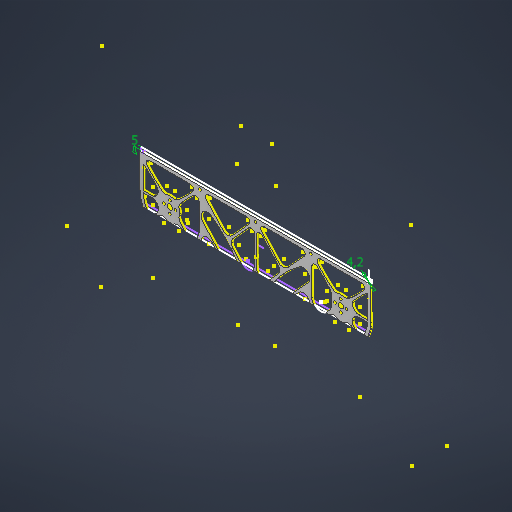
# Autodesk Inventor part: кб 2025-2026
Saved by Autodesk Inventor 2025 (Build 290162000, 162)
## iProperties
Created: 2025-09-02
Part Number: кб 2025-2026
Material: Типовые
Document SubType Name: Modeling
Designer: Phantom
Density: 1 g/cm^3
Appearance: По умолчанию
Author: Phantom
Autodesk Inventor part; units mm, degrees
(part 1 of 3)
ref_plane "YZ Plane" through (0, 0, 0) normal (1, 0, 0) x (0, 1, 0)
ref_plane "XZ Plane" through (0, 0, 0) normal (0, 1, 0) x (-1, 0, 0)
ref_plane "XY Plane" through (0, 0, 0) normal (0, 0, 1) x (1, 0, 0)
sketch "Эскиз1" plane through (0, 0, 0) normal (0, 0, 1) x (1, 0, 0)
  arc A0 (132.2862, -52.3121) -> (184.2862, -0.3121) centre (132.2862, -0.3121) ccw
  line L0 (-134.5611, -52.3121) -> (132.2862, -52.3121)
  line L1 (-186.5611, -0.3121) -> (-186.5611, 46.6879)
  line L2 (184.2862, -0.3121) -> (184.2862, 46.6879)
  line L3 (-134.5611, 51.6879) -> (-181.5611, 51.6879)
  line L4 (-181.5611, 51.6879) -> (179.2862, 51.6879)
  arc A1 (-186.5611, -0.3121) -> (-134.5611, -52.3121) centre (-134.5611, -0.3121) ccw
  circle A2 centre (-134.5611, -0.3121) radius 4
  circle A3 centre (-134.5611, 8.6879) radius 2.1
  circle A4 centre (-143.5611, -0.3121) radius 2.1
  circle A5 centre (-134.5611, -9.3121) radius 2.1
  circle A6 centre (-125.5611, -0.3121) radius 2.1
  circle A7 centre (132.2862, -0.3121) radius 4
  circle A8 centre (132.2862, 8.6879) radius 2.1
  circle A9 centre (123.2862, -0.3121) radius 2.1
  circle A10 centre (132.2862, -9.3121) radius 2.1
  circle A11 centre (141.2862, -0.3121) radius 2.1
  arc A12 (-181.5611, 51.6879) -> (-186.5611, 46.6879) centre (-181.5611, 46.6879) ccw
  arc A13 (184.2862, 46.6879) -> (179.2862, 51.6879) centre (179.2862, 46.6879) ccw
  circle A14 centre (-181.5611, 46.6879) radius 2.1
  circle A15 centre (179.2862, 46.6879) radius 2.1
  circle A16 centre (-87.5611, -47.3121) radius 2.1
  circle A17 centre (85.2862, -47.3121) radius 2.1
  circle A18 centre (-1.1374, -47.3121) radius 2.1
  circle A19 centre (-1.1374, 46.6879) radius 2.1
  circle A20 centre (-87.5611, 46.6879) radius 2.1
  circle A21 centre (85.2862, 46.6879) radius 2.1
  line L5 (179.2862, 44.5879) -> (179.2862, -0.3121)
  arc A22 (-181.5611, 51.6879) -> (-186.5611, 46.6879) centre (-181.5611, 46.6879) ccw
  line L6 (-181.5611, 44.5879) -> (-181.5611, -0.3121)
  arc A23 (-181.5611, -0.3121) -> (-134.5611, -47.3121) centre (-134.5611, -0.3121) ccw
  arc A24 (-164.0709, -36.8931) -> (-134.5611, -47.3121) centre (-134.5611, -0.3121) ccw
  arc A25 (-132.8051, -9.1391) -> (-132.4754, -9.0671) centre (-134.5611, -0.3121) ccw
  line L7 (-80.49, 46.6879) -> (-80.6353, 46.5425)
  line L8 (-174.49, 46.6879) -> (-89.6611, 46.6879)
  line L9 (-179.4611, 46.6879) -> (-94.6321, 46.6879)
  line L10 (-80.49, 46.6879) -> (-3.2374, 46.6879)
  line L11 (-85.4611, 46.6879) -> (-7.9295, 46.6879)
  line L12 (5.6547, 46.6879) -> (78.4941, 46.6879)
  line L13 (0.9626, 46.6879) -> (83.1862, 46.6879)
  line L14 (87.3862, 46.6879) -> (172.2152, 46.6879)
  line L15 (92.3573, 46.6879) -> (177.1862, 46.6879)
  arc A26 (132.2862, -47.3121) -> (179.2862, -0.3121) centre (132.2862, -0.3121) ccw
  arc A27 (168.8672, -29.822) -> (179.2862, -0.3121) centre (132.2862, -0.3121) ccw
  line L16 (-89.6611, -47.3121) -> (-134.5611, -47.3121)
  line L17 (-80.6353, -47.1668) -> (-80.49, -47.3121)
  line L18 (5.6547, -47.3121) -> (85.2862, -47.3121)
  line L19 (132.2862, -47.3121) -> (0.9626, -47.3121)
  line L20 (-7.9295, -47.3121) -> (-80.769, -47.3121)
  line L21 (-85.4611, -47.3121) -> (-3.2374, -47.3121)
  point P0 (-186.5611, 44.6168)
  point P1 (-75.49, 51.6879)
  point P2 (-1.1374, 46.6879)
  dimension "d2" = 8
  dimension "d4" = 4.2
  dimension "d7" = 360
  dimension "d13" = 4.2
  dimension "d14" = 360
  dimension "d15" = 5
  dimension "d17" = 4.2
  dimension "d19" = 4.2
  dimension "d21" = 4.2
  dimension "d23" = 4.2
  dimension "d35" = 99
  constraints: 44 end point, 35 point on circle, 27 centre point, 14 point on line, 10 tangent, 5 coincident, 1 equal radius, 1 horizontal, 1 vertical, 21 other
  measures "d2" diameter of A2
  measures "d4" diameter of A3
  measures "d13" diameter of A8
  measures "d15" radius of A12
  measures "d17" diameter of A14
  measures "d19" diameter of A15
  measures "d21" diameter of A16
  measures "d23" diameter of A19
  measures "d35" distance from line of L1 A16.centre
extrude "Выдавливание1" add sketch "Эскиз1" along normal blind 2 contours L0 A1 L1 A12 L3 L4 A13 L2 A0 | L9 L8 A20 L11 L10 A19 L13 L12 A21 L14 L15 A15 L5 A26 L19 A17 L18 A18 L21 L20 A16 L16 A23 L6 A14
sketch "Эскиз2" plane through (0, 0, 2) normal (0, 0, 1) x (1, 0, 0)
  arc A0 (-186.5611, -0.3121) -> (-134.5611, -52.3121) centre (-134.5611, -0.3121) ccw projected
  circle A1 centre (-143.5611, -0.3121) radius 2.1 projected
  circle A2 centre (-181.5611, 46.6879) radius 2.1 projected
  circle A3 centre (-87.5611, 46.6879) radius 2.1 projected
  line L0 (-181.5611, 46.6879) -> (-102.4688, 46.6879)
  circle A4 centre (-1.1374, -47.3121) radius 2.1 projected
  line L1 (-1.1374, -47.3121) -> (-87.5611, -47.3121)
  circle A5 centre (-134.5611, -0.3121) radius 15
  circle A6 centre (-87.5611, 46.6879) radius 5
  circle A7 centre (-181.5611, 46.6879) radius 5
  circle A8 centre (-87.5611, -47.3121) radius 5
  circle A9 centre (-1.1374, -47.3121) radius 5
  circle A10 centre (-1.1374, 46.6879) radius 5
  line L2 (179.2862, 51.6879) -> (-181.5611, 51.6879) projected
  arc A11 (-181.5611, 51.6879) -> (-186.5611, 46.6879) centre (-181.5611, 46.6879) ccw projected
  line L3 (-186.5611, 46.6879) -> (-186.5611, -0.3121) projected
  arc A12 (-186.5611, -0.3121) -> (-134.5611, -52.3121) centre (-134.5611, -0.3121) ccw projected
  line L4 (-134.5611, -52.3121) -> (132.2862, -52.3121) projected
  arc A13 (132.2862, -52.3121) -> (184.2862, -0.3121) centre (132.2862, -0.3121) ccw projected
  line L5 (184.2862, -0.3121) -> (184.2862, 46.6879) projected
  arc A14 (184.2862, 46.6879) -> (179.2862, 51.6879) centre (179.2862, 46.6879) ccw projected
  circle A15 centre (85.2862, -47.3121) radius 2.1 projected
  circle A16 centre (179.2862, 46.6879) radius 2.1 projected
  circle A17 centre (85.2862, 46.6879) radius 2.1 projected
  circle A18 centre (-1.1374, 46.6879) radius 2.1 projected
  circle A19 centre (-87.5611, 46.6879) radius 2.1 projected
  circle A20 centre (-181.5611, 46.6879) radius 2.1 projected
  circle A21 centre (-87.5611, -47.3121) radius 2.1 projected
  circle A22 centre (123.2862, -0.3121) radius 2.1 projected
  circle A23 centre (132.2862, 8.6879) radius 2.1 projected
  circle A24 centre (-125.5611, -0.3121) radius 2.1 projected
  circle A25 centre (-134.5611, -9.3121) radius 2.1 projected
  circle A26 centre (-134.5611, 8.6879) radius 2.1 projected
  circle A27 centre (-1.1374, -47.3121) radius 2.1 projected
  circle A28 centre (132.2862, -0.3121) radius 4 projected
  circle A29 centre (132.2862, -9.3121) radius 2.1 projected
  circle A30 centre (141.2862, -0.3121) radius 2.1 projected
  circle A31 centre (-143.5611, -0.3121) radius 2.1 projected
  circle A32 centre (-134.5611, -0.3121) radius 4 projected
  line L6 (179.2862, 46.6879) -> (179.2862, -0.3121)
  arc A33 (132.2862, -47.3121) -> (179.2862, -0.3121) centre (132.2862, -0.3121) ccw
  line L7 (-102.4787, -47.3121) -> (-128.0611, -47.3121)
  arc A34 (-180.9948, -7.5859) -> (-141.8349, -46.7458) centre (-134.5611, -0.3121) ccw
  line L8 (-181.5611, 6.1879) -> (-181.5611, 31.7702)
  line L9 (-88.1824, -48.8121) -> (-1.1374, -48.8121)
  line L10 (-180.0761, 45.203) -> (-181.5611, 46.6879)
  arc A35 (-181.5611, 6.1879) -> (-176.5611, 1.1879) centre (-176.5611, 6.1879) ccw
  arc A36 (-176.055, -1.8121) -> (-180.9948, -7.5859) centre (-176.055, -6.8121) ccw
  arc A37 (-141.8349, -46.7458) -> (-136.0611, -41.8061) centre (-141.0611, -41.8061) ccw
  arc A38 (-133.0611, -42.3121) -> (-128.0611, -47.3121) centre (-128.0611, -42.3121) ccw
  line L11 (85.2862, 46.6879) -> (85.2862, -47.3121)
  line L12 (85.2862, 46.6879) -> (-1.1374, -47.3121)
  line L13 (-87.5611, 41.6879) -> (-87.5611, -32.3944)
  line L14 (-133.0611, -15.2369) -> (-133.0611, -42.3121)
  line L15 (-134.5611, -15.3121) -> (-134.5611, -47.3121)
  line L16 (-136.0611, -15.2369) -> (-136.0611, -41.8061)
  line L17 (-149.4859, -1.8121) -> (-176.055, -1.8121)
  line L18 (-149.5611, -0.3121) -> (-181.5611, -0.3121)
  line L19 (-149.4859, 1.1879) -> (-176.5611, 1.1879)
  arc A39 (-126.2901, 12.2015) -> (-98.6785, 38.427) centre (-242.2895, 161.9803) ccw
  arc A40 (-97.3626, 34.2305) -> (-122.0474, 7.9589) centre (27.7313, -108.0406) ccw
  arc A41 (-147.0747, 7.9589) -> (-173.2978, 35.5585) centre (-297.8894, -109.0766) ccw
  arc A42 (-170.4316, 38.4246) -> (-142.832, 12.2015) centre (-25.7966, 163.0162) ccw
  arc A43 (-98.6905, -39.0488) -> (-126.2901, -12.8257) centre (-243.3255, -163.6405) ccw
  arc A44 (-122.0474, -8.5831) -> (-97.3647, -34.8414) centre (28.7673, 108.4524) ccw
  arc A45 (-166.6434, 46.6879) -> (-170.4316, 38.4246) centre (-166.6434, 41.6879) ccw
  arc A46 (-98.6785, 38.427) -> (-102.4688, 46.6879) centre (-102.4688, 41.6879) ccw
  arc A47 (-173.2978, 35.5585) -> (-181.5611, 31.7702) centre (-176.5611, 31.7702) ccw
  arc A48 (-102.4787, -47.3121) -> (-98.6905, -39.0488) centre (-102.4787, -42.3121) ccw
  line L20 (-84.177, 43.0071) -> (-1.1374, -47.3121)
  line L21 (-87.5611, 46.6879) -> (-85.4611, 46.6879)
  line L22 (-82.5611, 46.6879) -> (-14.5641, 46.6879)
  line L23 (-166.6434, 46.6879) -> (-85.4611, 46.6879)
  line L24 (-77.3803, 33.3984) -> (-12.2625, -37.428)
  line L25 (-77.8151, 38.3038) -> (-11.3182, -34.0226)
  line L26 (-87.5611, -47.3121) -> (-87.5611, -45.2121)
  line L27 (-87.5611, -42.3121) -> (-87.5611, 31.6458)
  line L28 (-86.9397, -45.8121) -> (-86.0914, -45.8121)
  line L29 (-82.7914, -45.8121) -> (-15.9432, -45.8121)
  arc A49 (-15.9432, -45.8121) -> (-12.2625, -37.428) centre (-15.9432, -40.8121) ccw
  line L30 (-89.0611, 30.4755) -> (-89.0611, -31.0883)
  line L31 (-86.0611, 30.0143) -> (-86.0611, -32.3944)
  arc A50 (-89.0611, 30.4755) -> (-97.3626, 34.2305) centre (-94.0611, 30.4755) ccw
  arc A51 (-97.3647, -34.8414) -> (-89.0611, -31.0883) centre (-94.0611, -31.0883) ccw
  arc A52 (-77.3803, 33.3984) -> (-86.0611, 30.0143) centre (-81.0611, 30.0143) ccw
  arc A53 (-86.0611, -1.1901) -> (-86.4175, -1.8121) centre (-59.5558, -16.7923) ccw
  arc A54 (-86.0611, -32.3944) -> (-69.7443, -45.8121) centre (-59.5558, -16.7923) ccw
  line L32 (-1.1374, 46.6879) -> (-2.5587, 45.142)
  line L33 (-4.5215, 43.0071) -> (-43.3304, 0.796)
  line L34 (-1.1374, 46.6879) -> (0.2839, 45.142)
  line L35 (2.2467, 43.0071) -> (42.0744, -0.3121)
  line L36 (-11.3182, 33.3984) -> (-42.3116, -0.3121)
  line L37 (9.0433, 33.3984) -> (40.9702, -1.3273)
  line L38 (8.6085, 38.3038) -> (43.1786, 0.7031)
  line L39 (-0.0332, -48.3273) -> (75.1055, 33.3984)
  line L40 (83.7862, 30.0143) -> (83.7862, -47.3121)
  line L41 (86.7862, 46.6879) -> (86.7862, -47.3121)
  line L42 (-1.1374, 46.6879) -> (-1.1374, 44.5879)
  line L43 (-1.1374, 41.6879) -> (-1.1374, -32.27)
  line L44 (-2.6374, 30.0143) -> (-2.6374, -30.6385)
  line L45 (0.3626, 30.0143) -> (0.3626, -30.6385)
  arc A55 (-11.3182, -34.0226) -> (-2.6374, -30.6385) centre (-7.6374, -30.6385) ccw
  arc A56 (0.3626, -30.6385) -> (9.0433, -34.0226) centre (5.3626, -30.6385) ccw
  line L46 (-10.8834, 38.3038) -> (-44.3492, 1.9041)
  line L47 (-45.368, 0.796) -> (-45.4535, 0.7031)
  arc A57 (-74.1343, 46.6879) -> (-77.8151, 38.3038) centre (-74.1343, 41.6879) ccw
  arc A58 (-10.8834, 38.3038) -> (-14.5641, 46.6879) centre (-14.5641, 41.6879) ccw
  arc A59 (12.2893, 46.6879) -> (8.6085, 38.3038) centre (12.2893, 41.6879) ccw
  arc A60 (-2.6374, 30.0143) -> (-11.3182, 33.3984) centre (-7.6374, 30.0143) ccw
  arc A61 (9.0433, 33.3984) -> (0.3626, 30.0143) centre (5.3626, 30.0143) ccw
  arc A62 (132.2862, -52.3121) -> (184.2862, -0.3121) centre (132.2862, -0.3121) ccw
  circle A63 centre (141.2862, -0.3121) radius 2.1
  circle A64 centre (179.2862, 46.6879) radius 2.1
  line L48 (179.2862, 46.6879) -> (100.194, 46.6879)
  circle A65 centre (132.2862, -0.3121) radius 15
  circle A66 centre (179.2862, 46.6879) radius 5
  arc A67 (184.2862, 46.6879) -> (179.2862, 51.6879) centre (179.2862, 46.6879) ccw
  line L49 (184.2862, 46.6879) -> (184.2862, -0.3121)
  arc A68 (132.2862, -52.3121) -> (184.2862, -0.3121) centre (132.2862, -0.3121) ccw
  circle A69 centre (179.2862, 46.6879) radius 2.1
  circle A70 centre (123.2862, -0.3121) radius 2.1
  circle A71 centre (132.2862, -9.3121) radius 2.1
  circle A72 centre (132.2862, 8.6879) radius 2.1
  circle A73 centre (141.2862, -0.3121) radius 2.1
  circle A74 centre (132.2862, -0.3121) radius 4
  line L50 (100.2039, -47.3121) -> (125.7862, -47.3121)
  arc A75 (139.56, -46.7458) -> (178.72, -7.5859) centre (132.2862, -0.3121) ccw
  line L51 (179.2862, 6.1879) -> (179.2862, 31.7702)
  line L52 (177.8013, 45.203) -> (179.2862, 46.6879)
  arc A76 (174.2862, 1.1879) -> (179.2862, 6.1879) centre (174.2862, 6.1879) ccw
  arc A77 (178.72, -7.5859) -> (173.7802, -1.8121) centre (173.7802, -6.8121) ccw
  arc A78 (133.7862, -41.8061) -> (139.56, -46.7458) centre (138.7862, -41.8061) ccw
  arc A79 (125.7862, -47.3121) -> (130.7862, -42.3121) centre (125.7862, -42.3121) ccw
  line L53 (85.2862, 41.6879) -> (85.2862, -32.3944)
  line L54 (130.7862, -15.2369) -> (130.7862, -42.3121)
  line L55 (132.2862, -15.3121) -> (132.2862, -47.3121)
  line L56 (133.7862, -15.2369) -> (133.7862, -41.8061)
  line L57 (147.211, -1.8121) -> (173.7802, -1.8121)
  line L58 (147.2862, -0.3121) -> (179.2862, -0.3121)
  line L59 (147.211, 1.1879) -> (174.2862, 1.1879)
  arc A80 (96.4037, 38.427) -> (124.0152, 12.2015) centre (240.0147, 161.9803) ccw
  arc A81 (119.7726, 7.9589) -> (95.0878, 34.2305) centre (-30.0061, -108.0406) ccw
  arc A82 (171.0229, 35.5585) -> (144.7998, 7.9589) centre (295.6146, -109.0766) ccw
  arc A83 (140.5572, 12.2015) -> (168.1568, 38.4246) centre (23.5217, 163.0162) ccw
  arc A84 (95.0899, -34.8414) -> (119.7726, -8.5831) centre (-31.0421, 108.4524) ccw
  arc A85 (124.0152, -12.8257) -> (96.4156, -39.0488) centre (241.0507, -163.6405) ccw
  arc A86 (168.1568, 38.4246) -> (164.3686, 46.6879) centre (164.3686, 41.6879) ccw
  arc A87 (100.194, 46.6879) -> (96.4037, 38.427) centre (100.194, 41.6879) ccw
  arc A88 (179.2862, 31.7702) -> (171.0229, 35.5585) centre (174.2862, 31.7702) ccw
  arc A89 (96.4156, -39.0488) -> (100.2039, -47.3121) centre (100.2039, -42.3121) ccw
  line L60 (85.2862, -47.3121) -> (85.2862, -45.2121)
  line L61 (85.2862, -42.3121) -> (85.2862, 31.6458)
  line L62 (84.6649, -45.8121) -> (83.8165, -45.8121)
  line L63 (86.7862, 30.4755) -> (86.7862, -31.0883)
  line L64 (83.7862, 30.0143) -> (83.7862, -32.3944)
  arc A90 (95.0878, 34.2305) -> (86.7862, 30.4755) centre (91.7862, 30.4755) ccw
  arc A91 (86.7862, -31.0883) -> (95.0899, -34.8414) centre (91.7862, -31.0883) ccw
  arc A92 (84.1427, -1.8121) -> (83.7862, -1.1901) centre (57.281, -16.7923) ccw
  circle A93 centre (-1.1374, -47.3121) radius 2.1
  line L65 (-1.1374, -47.3121) -> (85.2862, -47.3121)
  circle A94 centre (-1.1374, -47.3121) radius 2.1
  line L66 (85.9075, -48.8121) -> (-1.1374, -48.8121)
  arc A95 (86.7862, -31.0883) -> (95.0899, -34.8414) centre (91.7862, -31.0883) ccw
  arc A96 (9.9876, -37.428) -> (13.6684, -45.8121) centre (13.6684, -40.8121) ccw
  line L67 (80.5165, -45.8121) -> (13.6684, -45.8121)
  arc A97 (67.4694, -45.8121) -> (83.7862, -32.3944) centre (57.281, -16.7923) ccw
  arc A98 (75.5403, 38.3038) -> (71.8595, 46.6879) centre (71.8595, 41.6879) ccw
  line L68 (12.2893, 46.6879) -> (71.8595, 46.6879)
  line L69 (83.1862, 46.6879) -> (179.2862, 46.6879)
  line L70 (9.0433, -34.0226) -> (75.5403, 38.3038)
  line L71 (83.1873, 46.6212) -> (83.2486, 46.6879)
  arc A99 (83.7862, 30.0143) -> (75.1055, 33.3984) centre (78.7862, 30.0143) ccw
  point P0 (0, 0)
  point P1 (-177.1277, 44.3759)
  point P2 (-181.5611, 41.6879)
  point P3 (-92.5611, -47.3121)
  point P4 (-92.5611, 46.6879)
  point P5 (-176.5611, 46.6879)
  point P6 (-82.5611, -47.3121)
  point P7 (-82.7914, -48.8121)
  point P8 (-144.0538, 11.302)
  point P9 (-82.5611, -47.3121)
  point P10 (-6.1374, -47.3121)
  point P11 (-88.2682, 41.7381)
  point P12 (-122.0474, 7.9589)
  point P13 (-87.5611, 41.6879)
  point P14 (-122.0474, -8.5831)
  point P15 (-88.2682, -42.3624)
  point P16 (-92.5108, -46.605)
  point P17 (-126.2901, -12.8257)
  point P18 (-89.0611, -41.7437)
  point P19 (-83.2286, 44.1919)
  point P20 (-5.4699, 44.1919)
  point P21 (-3.2614, 42.1614)
  point P22 (0.9866, 42.1614)
  point P23 (3.195, 44.1919)
  point P24 (-2.6374, 41.9182)
  point P25 (0.3626, 41.9182)
  point P26 (-6.1374, 46.6879)
  point P27 (-74.1343, 46.6879)
  point P28 (85.2862, -47.3121)
  point P29 (85.2862, -47.3121)
  point P30 (85.2862, 46.6879)
  point P31 (85.9075, -48.8121)
  point P32 (174.8529, 44.3759)
  point P33 (141.779, 11.302)
  point P34 (86.7862, -41.7437)
  point P35 (-2.2416, -48.3273)
  point P36 (139.56, -46.7458)
  point P37 (178.72, -7.5859)
  point P38 (124.0152, -12.8257)
  point P39 (119.7726, -8.5831)
  point P40 (119.7726, 7.9589)
  point P41 (67.4694, -45.8121)
  point P42 (42.0744, 1.9041)
  point P43 (40.0368, -0.3121)
  dimension "d44" = 30
  dimension "d46" = 10
  dimension "d49" = 10
  dimension "d45" = 10
  dimension "d47" = 10
  dimension "d48" = 10
  dimension "d60" = 5
  dimension "d61" = 5
  dimension "d66" = 5
  dimension "d67" = 1.5
  dimension "d68" = 1.5
  dimension "d70" = 5
  dimension "d71" = 1.5
  dimension "d72" = 1.5
  dimension "d73" = 5
  dimension "d74" = 5
  dimension "d76" = 1.5
  dimension "d77" = 1.5
  dimension "d78" = 1.5
  dimension "d79" = 1.5
  dimension "d82" = 1.5
  dimension "d83" = 1.5
  dimension "d84" = 5
  dimension "d86" = 5
  constraints: 136 end point, 129 point on circle, 103 symmetric about line, 67 centre point, 43 tangent, 33 point on line, 17 parallel, 11 coincident, 9 equal radius, 8 perpendicular, 4 vertical, 2 midpoint, 1 horizontal, 1 horizontal alignment, 86 other
  measures "d45" diameter of A6
  measures "d47" diameter of A8
  measures "d48" diameter of A9
  measures "d60" radius of A35
  measures "d61" radius of A36
  measures "d66" radius of A45
  measures "d67" distance between parallel lines of L20 L24
  measures "d68" distance between parallel lines of L20 L25
  measures "d70" radius of A49
  measures "d71" distance between parallel lines of L13 L30
  measures "d72" distance between parallel lines of L13 L31
  measures "d73" radius of A50
  measures "d74" radius of A51
  measures "d76" distance between parallel lines of L33 L36
  measures "d77" distance between parallel lines of L35 L37
  measures "d78" distance between parallel lines of L35 L38
  measures "d79" distance between parallel lines of L12 L39
  measures "d82" distance between parallel lines of L43 L44
  measures "d83" distance between parallel lines of L43 L45
  measures "d84" radius of A55
  measures "d86" radius of A57
extrude "Выдавливание2" cut sketch "Эскиз2" against normal blind 2 contours L0 A46 A39 A5 A42 A45 | L38 A59 L68 A98 L70 | L22 A58 L46 L25 A57 | A5 L19 A35 L8 A47 A41 | L39 A99 L40 A97 L67 A96 | A86 A83 A65 A80 A87 L48 | A40 A50 L30 A51 A44 A5 | L41 A90 A81 A65 A84 A91 | L6 A76 L59 A65 A82 A88 | L69 A17 | A17 L41 L69 | A5 L16 A37 A34 A36 L17 | L12 L11 A17 | A17 L71 L69 L12 | A17 L11 L69 L41 | L69 L71 A17 | A43 A48 L7 A38 L14 A5 | A65 L54 A79 L50 A89 A85 | A33 A78 L56 A65 L57 A77 | L24 A49 L29 A54 L31 A52 | L36 A60 L44 A55 L25 | L37 L70 A56 L45 A61
fillet "Сопряжение1" radius 10 23 edges at (-126.2901, 12.2015, 1) (-122.0474, 7.9589, 1) (-142.832, 12.2015, 1) (-147.0747, 7.9589, 1) (-122.0474, -8.5831, 1) (-126.2901, -12.8257, 1) (-133.0611, -15.2369, 1) (-136.0611, -15.2369, 1) (-149.4859, -1.8121, 1) (-149.4859, 1.1879, 1) (-44.3492, 1.9041, 1) (-42.3116, -0.3121, 1) (40.0368, -0.3121, 1) (133.7862, -15.2369, 1) (147.211, -1.8121, 1) (130.7862, -15.2369, 1) (124.0152, -12.8257, 1) (144.7998, 7.9589, 1) (147.211, 1.1879, 1) (119.7726, 7.9589, 1) (119.7726, -8.5831, 1) (140.5572, 12.2015, 1) (124.0152, 12.2015, 1)
sketch "Эскиз3" plane through (0, 0, 2) normal (0, 0, 1) x (1, 0, 0)
  point P0 (0, 0)
sketch "Эскиз4" plane through (0, 0, 2) normal (0, 0, 1) x (1, 0, 0)
  line L0 (-162.7567, 1.1879) -> (-176.5611, 1.1879) projected
  arc A0 (-181.5611, 6.1879) -> (-176.5611, 1.1879) centre (-176.5611, 6.1879) ccw projected
  line L1 (-181.5611, 6.1879) -> (-181.5611, 31.7702) projected
  arc A1 (-173.2978, 35.5585) -> (-181.5611, 31.7702) centre (-176.5611, 31.7702) ccw projected
  arc A2 (-155.2866, 17.836) -> (-173.2978, 35.5585) centre (-297.8894, -109.0766) ccw projected
  arc A3 (-162.7567, 1.1879) -> (-155.2866, 17.836) centre (-162.7567, 11.1879) ccw projected
  arc A4 (9.9876, -37.428) -> (13.6684, -45.8121) centre (13.6684, -40.8121) ccw projected
  line L2 (9.9876, -37.428) -> (75.1055, 33.3984) projected
  arc A5 (83.7862, 30.0143) -> (75.1055, 33.3984) centre (78.7862, 30.0143) ccw projected
  line L3 (83.7862, 30.0143) -> (83.7862, -32.3944) projected
  arc A6 (67.4694, -45.8121) -> (83.7862, -32.3944) centre (57.281, -16.7923) ccw projected
  line L4 (67.4694, -45.8121) -> (13.6684, -45.8121) projected
  arc A7 (136.3136, 14.1371) -> (128.2552, 14.1361) centre (132.2862, -0.3121) ccw projected
  arc A8 (119.19, 16.0661) -> (128.2552, 14.1361) centre (125.5679, 23.7682) ccw projected
  arc A9 (96.4037, 38.427) -> (119.19, 16.0661) centre (240.0147, 161.9803) ccw projected
  arc A10 (100.194, 46.6879) -> (96.4037, 38.427) centre (100.194, 41.6879) ccw projected
  line L5 (100.194, 46.6879) -> (164.3686, 46.6879) projected
  arc A11 (168.1568, 38.4246) -> (164.3686, 46.6879) centre (164.3686, 41.6879) ccw projected
  arc A12 (145.382, 16.0725) -> (168.1568, 38.4246) centre (23.5217, 163.0162) ccw projected
  arc A13 (136.3136, 14.1371) -> (145.382, 16.0725) centre (138.9985, 23.7699) ccw projected
  line L6 (9.0433, 33.3984) -> (33.8141, 6.4561) projected
  arc A14 (33.8141, -7.0803) -> (33.8141, 6.4561) centre (26.4526, -0.3121) ccw projected
  line L7 (33.8141, -7.0803) -> (9.0433, -34.0226) projected
  arc A15 (0.3626, -30.6385) -> (9.0433, -34.0226) centre (5.3626, -30.6385) ccw projected
  line L8 (0.3626, -30.6385) -> (0.3626, 30.0143) projected
  arc A16 (9.0433, 33.3984) -> (0.3626, 30.0143) centre (5.3626, 30.0143) ccw projected
  arc A17 (-166.6434, 46.6879) -> (-170.4316, 38.4246) centre (-166.6434, 41.6879) ccw projected
  line L9 (-166.6434, 46.6879) -> (-102.4688, 46.6879) projected
  arc A18 (-98.6785, 38.427) -> (-102.4688, 46.6879) centre (-102.4688, 41.6879) ccw projected
  arc A19 (-121.4649, 16.0661) -> (-98.6785, 38.427) centre (-242.2895, 161.9803) ccw projected
  arc A20 (-130.53, 14.1361) -> (-121.4649, 16.0661) centre (-127.8427, 23.7682) ccw projected
  arc A21 (-130.53, 14.1361) -> (-138.5884, 14.1371) centre (-134.5611, -0.3121) ccw projected
  arc A22 (-147.6568, 16.0725) -> (-138.5884, 14.1371) centre (-141.2733, 23.7699) ccw projected
  arc A23 (-170.4316, 38.4246) -> (-147.6568, 16.0725) centre (-25.7966, 163.0162) ccw projected
  arc A24 (-86.0611, -32.3944) -> (-69.7443, -45.8121) centre (-59.5558, -16.7923) ccw projected
  line L10 (-86.0611, -32.3944) -> (-86.0611, 30.0143) projected
  arc A25 (-77.3803, 33.3984) -> (-86.0611, 30.0143) centre (-81.0611, 30.0143) ccw projected
  line L11 (-77.3803, 33.3984) -> (-12.2625, -37.428) projected
  arc A26 (-15.9432, -45.8121) -> (-12.2625, -37.428) centre (-15.9432, -40.8121) ccw projected
  line L12 (-15.9432, -45.8121) -> (-69.7443, -45.8121) projected
  arc A27 (133.7862, -41.8061) -> (139.56, -46.7458) centre (138.7862, -41.8061) ccw projected
  line L13 (133.7862, -41.8061) -> (133.7862, -22.5101) projected
  arc A28 (139.1862, -13.6309) -> (133.7862, -22.5101) centre (143.7862, -22.5101) ccw projected
  arc A29 (139.1862, -13.6309) -> (145.605, -7.2121) centre (132.2862, -0.3121) ccw projected
  arc A30 (154.4842, -1.8121) -> (145.605, -7.2121) centre (154.4842, -11.8121) ccw projected
  line L14 (154.4842, -1.8121) -> (173.7802, -1.8121) projected
  arc A31 (178.72, -7.5859) -> (173.7802, -1.8121) centre (173.7802, -6.8121) ccw projected
  arc A32 (139.56, -46.7458) -> (178.72, -7.5859) centre (132.2862, -0.3121) ccw projected
  arc A33 (95.0878, 34.2305) -> (86.7862, 30.4755) centre (91.7862, 30.4755) ccw projected
  arc A34 (115.908, 12.7841) -> (95.0878, 34.2305) centre (-30.0061, -108.0406) ccw projected
  arc A35 (117.838, 3.7189) -> (115.908, 12.7841) centre (108.2059, 6.4063) ccw projected
  arc A36 (117.838, 3.7189) -> (117.837, -4.3395) centre (132.2862, -0.3121) ccw projected
  arc A37 (115.9016, -13.4079) -> (117.837, -4.3395) centre (108.2042, -7.0244) ccw projected
  arc A38 (95.0899, -34.8414) -> (115.9016, -13.4079) centre (-31.0421, 108.4524) ccw projected
  arc A39 (86.7862, -31.0883) -> (95.0899, -34.8414) centre (91.7862, -31.0883) ccw projected
  line L15 (86.7862, -31.0883) -> (86.7862, 30.4755) projected
  arc A40 (174.2862, 1.1879) -> (179.2862, 6.1879) centre (174.2862, 6.1879) ccw projected
  line L16 (174.2862, 1.1879) -> (160.4818, 1.1879) projected
  arc A41 (153.0118, 17.836) -> (160.4818, 1.1879) centre (160.4818, 11.1879) ccw projected
  arc A42 (171.0229, 35.5585) -> (153.0118, 17.836) centre (295.6146, -109.0766) ccw projected
  arc A43 (179.2862, 31.7702) -> (171.0229, 35.5585) centre (174.2862, 31.7702) ccw projected
  line L17 (179.2862, 31.7702) -> (179.2862, 6.1879) projected
  line L18 (-11.3182, -34.0226) -> (-36.0889, -7.0803) projected
  arc A44 (-36.0889, 6.4561) -> (-36.0889, -7.0803) centre (-28.7274, -0.3121) ccw projected
  line L19 (-36.0889, 6.4561) -> (-11.3182, 33.3984) projected
  arc A45 (-2.6374, 30.0143) -> (-11.3182, 33.3984) centre (-7.6374, 30.0143) ccw projected
  line L20 (-2.6374, 30.0143) -> (-2.6374, -30.6385) projected
  arc A46 (-11.3182, -34.0226) -> (-2.6374, -30.6385) centre (-7.6374, -30.6385) ccw projected
  arc A47 (-147.8798, -7.2121) -> (-141.4611, -13.6309) centre (-134.5611, -0.3121) ccw projected
  arc A48 (-136.0611, -22.5101) -> (-141.4611, -13.6309) centre (-146.0611, -22.5101) ccw projected
  line L21 (-136.0611, -22.5101) -> (-136.0611, -41.8061) projected
  arc A49 (-141.8349, -46.7458) -> (-136.0611, -41.8061) centre (-141.0611, -41.8061) ccw projected
  arc A50 (-180.9948, -7.5859) -> (-141.8349, -46.7458) centre (-134.5611, -0.3121) ccw projected
  arc A51 (-176.055, -1.8121) -> (-180.9948, -7.5859) centre (-176.055, -6.8121) ccw projected
  line L22 (-176.055, -1.8121) -> (-156.759, -1.8121) projected
  arc A52 (-147.8798, -7.2121) -> (-156.759, -1.8121) centre (-156.759, -11.8121) ccw projected
  arc A53 (-120.1118, -4.3395) -> (-120.1128, 3.7189) centre (-134.5611, -0.3121) ccw projected
  arc A54 (-118.1829, 12.7841) -> (-120.1128, 3.7189) centre (-110.4807, 6.4063) ccw projected
  arc A55 (-97.3626, 34.2305) -> (-118.1829, 12.7841) centre (27.7313, -108.0406) ccw projected
  arc A56 (-89.0611, 30.4755) -> (-97.3626, 34.2305) centre (-94.0611, 30.4755) ccw projected
  line L23 (-89.0611, 30.4755) -> (-89.0611, -31.0883) projected
  arc A57 (-97.3647, -34.8414) -> (-89.0611, -31.0883) centre (-94.0611, -31.0883) ccw projected
  arc A58 (-118.1765, -13.4079) -> (-97.3647, -34.8414) centre (28.7673, 108.4524) ccw projected
  arc A59 (-120.1118, -4.3395) -> (-118.1765, -13.4079) centre (-110.479, -7.0244) ccw projected
  arc A60 (-102.4787, -47.3121) -> (-98.6905, -39.0488) centre (-102.4787, -42.3121) ccw projected
  line L24 (-102.4787, -47.3121) -> (-128.0611, -47.3121) projected
  arc A61 (-133.0611, -42.3121) -> (-128.0611, -47.3121) centre (-128.0611, -42.3121) ccw projected
  line L25 (-133.0611, -42.3121) -> (-133.0611, -28.5077) projected
  arc A62 (-116.4129, -21.0376) -> (-133.0611, -28.5077) centre (-123.0611, -28.5077) ccw projected
  arc A63 (-98.6905, -39.0488) -> (-116.4129, -21.0376) centre (-243.3255, -163.6405) ccw projected
  arc A64 (-74.1343, 46.6879) -> (-77.8151, 38.3038) centre (-74.1343, 41.6879) ccw projected
  line L26 (-74.1343, 46.6879) -> (-14.5641, 46.6879) projected
  arc A65 (-10.8834, 38.3038) -> (-14.5641, 46.6879) centre (-14.5641, 41.6879) ccw projected
  line L27 (-10.8834, 38.3038) -> (-36.9877, 9.911) projected
  arc A66 (-51.7107, 9.911) -> (-36.9877, 9.911) centre (-44.3492, 16.6792) ccw projected
  line L28 (-51.7107, 9.911) -> (-77.8151, 38.3038) projected
  arc A67 (130.7862, -28.5077) -> (114.1381, -21.0376) centre (120.7862, -28.5077) ccw projected
  line L29 (130.7862, -28.5077) -> (130.7862, -42.3121) projected
  arc A68 (125.7862, -47.3121) -> (130.7862, -42.3121) centre (125.7862, -42.3121) ccw projected
  line L30 (125.7862, -47.3121) -> (100.2039, -47.3121) projected
  arc A69 (96.4156, -39.0488) -> (100.2039, -47.3121) centre (100.2039, -42.3121) ccw projected
  arc A70 (114.1381, -21.0376) -> (96.4156, -39.0488) centre (241.0507, -163.6405) ccw projected
  line L31 (75.5403, 38.3038) -> (42.0744, 1.9041) projected
  line L32 (42.0744, 1.9041) -> (8.6085, 38.3038) projected
  arc A71 (12.2893, 46.6879) -> (8.6085, 38.3038) centre (12.2893, 41.6879) ccw projected
  line L33 (12.2893, 46.6879) -> (71.8595, 46.6879) projected
  arc A72 (75.5403, 38.3038) -> (71.8595, 46.6879) centre (71.8595, 41.6879) ccw projected
  line L34 (179.2862, 51.6879) -> (-181.5611, 51.6879) projected
  arc A73 (-181.5611, 51.6879) -> (-186.5611, 46.6879) centre (-181.5611, 46.6879) ccw projected
  line L35 (-186.5611, 46.6879) -> (-186.5611, -0.3121) projected
  arc A74 (-186.5611, -0.3121) -> (-134.5611, -52.3121) centre (-134.5611, -0.3121) ccw projected
  line L36 (-134.5611, -52.3121) -> (132.2862, -52.3121) projected
  arc A75 (132.2862, -52.3121) -> (184.2862, -0.3121) centre (132.2862, -0.3121) ccw projected
  line L37 (184.2862, -0.3121) -> (184.2862, 46.6879) projected
  arc A76 (184.2862, 46.6879) -> (179.2862, 51.6879) centre (179.2862, 46.6879) ccw projected
  circle A77 centre (85.2862, -47.3121) radius 2.1 projected
  circle A78 centre (179.2862, 46.6879) radius 2.1 projected
  circle A79 centre (85.2862, 46.6879) radius 2.1 projected
  circle A80 centre (-1.1374, 46.6879) radius 2.1 projected
  circle A81 centre (-87.5611, 46.6879) radius 2.1 projected
  circle A82 centre (-181.5611, 46.6879) radius 2.1 projected
  circle A83 centre (-87.5611, -47.3121) radius 2.1 projected
  circle A84 centre (123.2862, -0.3121) radius 2.1 projected
  circle A85 centre (132.2862, 8.6879) radius 2.1 projected
  circle A86 centre (-125.5611, -0.3121) radius 2.1 projected
  circle A87 centre (-134.5611, -9.3121) radius 2.1 projected
  circle A88 centre (-134.5611, 8.6879) radius 2.1 projected
  circle A89 centre (-1.1374, -47.3121) radius 2.1 projected
  circle A90 centre (132.2862, -0.3121) radius 4 projected
  circle A91 centre (132.2862, -9.3121) radius 2.1 projected
  circle A92 centre (141.2862, -0.3121) radius 2.1 projected
  circle A93 centre (-143.5611, -0.3121) radius 2.1 projected
  circle A94 centre (-134.5611, -0.3121) radius 4 projected
  line L38 (-134.5611, -0.3121) -> (-167.7951, -33.5461)
  line L39 (-135.6217, 0.7485) -> (-168.8557, -32.4855)
  line L40 (-133.5004, -1.3728) -> (-166.7344, -34.6068)
  line L41 (-1.1374, 46.6879) -> (-1.1374, -47.3121)
  line L42 (132.2862, -0.3121) -> (165.5202, -33.5461)
  line L43 (133.3469, 0.7485) -> (166.5809, -32.4855)
  line L44 (131.2256, -1.3728) -> (164.4596, -34.6068)
  point P0 (0, 0)
  point P1 (-166.7175, -34.5899)
  point P2 (-144.0538, -11.9262)
  point P3 (-146.1751, -9.8049)
  point P4 (-168.8388, -32.4685)
  point P5 (166.564, -32.4685)
  point P6 (143.9003, -9.8049)
  point P7 (141.779, -11.9262)
  point P8 (164.4426, -34.5899)
  dimension "d87" = 1.5
  dimension "d88" = 1.5
  constraints: 14 end point, 6 symmetric about line, 2 parallel, 1 point on circle, 1 vertical
  measures "d87" distance between parallel lines of L38 L39
  measures "d88" distance between parallel lines of L38 L40
extrude "Выдавливание3" add sketch "Эскиз4" against normal blind 2 contours L44 A29 L42 A32 | L42 A29 L43 A32 | A47 L38 A50 L39 | A47 L40 A50 L38
fillet "Сопряжение3" radius 10 8 edges at (-146.1751, -9.8049, 1) (-144.0538, -11.9262, 1) (-166.7175, -34.5899, 1) (-168.8388, -32.4685, 1) (166.564, -32.4685, 1) (143.9003, -9.8049, 1) (164.4426, -34.5899, 1) (141.779, -11.9262, 1)
sketch "Эскиз5" plane through (0, 0, 2) normal (0, 0, 1) x (1, 0, 0)
  line L0 (-86.0611, 30.0143) -> (-86.0611, -32.3944) projected
  line L1 (-69.7443, -45.8121) -> (-15.9432, -45.8121) projected
  arc A0 (-86.0611, -1.1901) -> (-63, -45.8121) centre (-20.9903, 4.1689) ccw
  arc A1 (-86.0611, -32.3944) -> (-69.7443, -45.8121) centre (-59.5558, -16.7923) ccw projected
  circle A2 centre (-1.1374, 46.6879) radius 2.1 projected
  circle A3 centre (-1.1374, -47.3121) radius 2.1 projected
  line L2 (-1.1374, 46.6879) -> (-1.1374, -47.3121)
  line L3 (83.7862, 30.0143) -> (83.7862, -32.3944)
  line L4 (67.4694, -45.8121) -> (13.6684, -45.8121)
  arc A4 (60.7252, -45.8121) -> (83.7862, -1.1901) centre (18.7155, 4.1689) ccw
  arc A5 (67.4694, -45.8121) -> (83.7862, -32.3944) centre (57.281, -16.7923) ccw
  point P0 (0, 0)
  constraints: 8 symmetric about line, 6 end point, 6 point on circle, 3 centre point, 2 point on line, 1 midpoint, 1 vertical, 2 other
sketch "Эскиз6" plane through (0, 0, 2) normal (0, 0, 1) x (1, 0, 0)
  line L0 (-77.3803, 33.3984) -> (-12.2625, -37.428) projected
  line L1 (-95.7841, 16.4779) -> (-30.6662, -54.3485)
  line L2 (-94.6798, 17.4932) -> (-29.562, -53.3332)
  line L3 (-96.8883, 15.4627) -> (-31.7705, -55.3637)
  circle A0 centre (-1.1374, 46.6879) radius 2.1 projected
  circle A1 centre (-1.1374, -47.3121) radius 2.1 projected
  line L4 (-1.1374, 46.6879) -> (-1.1374, -47.3121)
  line L5 (93.5092, 16.4779) -> (28.3914, -54.3485)
  line L6 (92.405, 17.4932) -> (27.2872, -53.3332)
  line L7 (94.6135, 15.4627) -> (29.4956, -55.3637)
  arc A2 (-180.9948, -7.5859) -> (-176.4785, -21.5706) centre (-134.5611, -0.3121) ccw projected
  arc A3 (-176.055, -1.8121) -> (-180.9948, -7.5859) centre (-176.055, -6.8121) ccw projected
  line L8 (-176.055, -1.8121) -> (-162.3245, -1.8121) projected
  arc A4 (-155.2534, -18.8832) -> (-162.3245, -1.8121) centre (-162.3245, -11.8121) ccw projected
  line L9 (-155.2534, -18.8832) -> (-160.4889, -24.1186) projected
  arc A5 (-176.4785, -21.5706) -> (-160.4889, -24.1186) centre (-167.5599, -17.0475) ccw projected
  arc A6 (139.56, -46.7458) -> (153.5447, -42.2296) centre (132.2862, -0.3121) ccw projected
  arc A7 (133.7862, -41.8061) -> (139.56, -46.7458) centre (138.7862, -41.8061) ccw projected
  line L10 (133.7862, -41.8061) -> (133.7862, -28.0756) projected
  arc A8 (150.8573, -21.0045) -> (133.7862, -28.0756) centre (143.7862, -28.0756) ccw projected
  line L11 (150.8573, -21.0045) -> (156.0927, -26.2399) projected
  arc A9 (153.5447, -42.2296) -> (156.0927, -26.2399) centre (149.0216, -33.311) ccw projected
  line L12 (-162.7567, 1.1879) -> (-176.5611, 1.1879) projected
  arc A10 (-181.5611, 6.1879) -> (-176.5611, 1.1879) centre (-176.5611, 6.1879) ccw projected
  line L13 (-181.5611, 6.1879) -> (-181.5611, 31.7702) projected
  arc A11 (-173.2978, 35.5585) -> (-181.5611, 31.7702) centre (-176.5611, 31.7702) ccw projected
  arc A12 (-155.2866, 17.836) -> (-173.2978, 35.5585) centre (-297.8894, -109.0766) ccw projected
  arc A13 (-162.7567, 1.1879) -> (-155.2866, 17.836) centre (-162.7567, 11.1879) ccw projected
  arc A14 (9.9876, -37.428) -> (13.6684, -45.8121) centre (13.6684, -40.8121) ccw projected
  line L14 (9.9876, -37.428) -> (75.1055, 33.3984) projected
  arc A15 (83.7862, 30.0143) -> (75.1055, 33.3984) centre (78.7862, 30.0143) ccw projected
  line L15 (83.7862, 30.0143) -> (83.7862, -32.3944) projected
  arc A16 (67.4694, -45.8121) -> (83.7862, -32.3944) centre (57.281, -16.7923) ccw projected
  line L16 (67.4694, -45.8121) -> (13.6684, -45.8121) projected
  arc A17 (136.3136, 14.1371) -> (128.2552, 14.1361) centre (132.2862, -0.3121) ccw projected
  arc A18 (119.19, 16.0661) -> (128.2552, 14.1361) centre (125.5679, 23.7682) ccw projected
  arc A19 (96.4037, 38.427) -> (119.19, 16.0661) centre (240.0147, 161.9803) ccw projected
  arc A20 (100.194, 46.6879) -> (96.4037, 38.427) centre (100.194, 41.6879) ccw projected
  line L17 (100.194, 46.6879) -> (164.3686, 46.6879) projected
  arc A21 (168.1568, 38.4246) -> (164.3686, 46.6879) centre (164.3686, 41.6879) ccw projected
  arc A22 (145.382, 16.0725) -> (168.1568, 38.4246) centre (23.5217, 163.0162) ccw projected
  arc A23 (136.3136, 14.1371) -> (145.382, 16.0725) centre (138.9985, 23.7699) ccw projected
  line L18 (9.0433, 33.3984) -> (33.8141, 6.4561) projected
  arc A24 (33.8141, -7.0803) -> (33.8141, 6.4561) centre (26.4526, -0.3121) ccw projected
  line L19 (33.8141, -7.0803) -> (9.0433, -34.0226) projected
  arc A25 (0.3626, -30.6385) -> (9.0433, -34.0226) centre (5.3626, -30.6385) ccw projected
  line L20 (0.3626, -30.6385) -> (0.3626, 30.0143) projected
  arc A26 (9.0433, 33.3984) -> (0.3626, 30.0143) centre (5.3626, 30.0143) ccw projected
  arc A27 (-166.6434, 46.6879) -> (-170.4316, 38.4246) centre (-166.6434, 41.6879) ccw projected
  line L21 (-166.6434, 46.6879) -> (-102.4688, 46.6879) projected
  arc A28 (-98.6785, 38.427) -> (-102.4688, 46.6879) centre (-102.4688, 41.6879) ccw projected
  arc A29 (-121.4649, 16.0661) -> (-98.6785, 38.427) centre (-242.2895, 161.9803) ccw projected
  arc A30 (-130.53, 14.1361) -> (-121.4649, 16.0661) centre (-127.8427, 23.7682) ccw projected
  arc A31 (-130.53, 14.1361) -> (-138.5884, 14.1371) centre (-134.5611, -0.3121) ccw projected
  arc A32 (-147.6568, 16.0725) -> (-138.5884, 14.1371) centre (-141.2733, 23.7699) ccw projected
  arc A33 (-170.4316, 38.4246) -> (-147.6568, 16.0725) centre (-25.7966, 163.0162) ccw projected
  arc A34 (-86.0611, -32.3944) -> (-69.7443, -45.8121) centre (-59.5558, -16.7923) ccw projected
  line L22 (-86.0611, -32.3944) -> (-86.0611, 30.0143) projected
  arc A35 (-77.3803, 33.3984) -> (-86.0611, 30.0143) centre (-81.0611, 30.0143) ccw projected
  line L23 (-77.3803, 33.3984) -> (-12.2625, -37.428) projected
  arc A36 (-15.9432, -45.8121) -> (-12.2625, -37.428) centre (-15.9432, -40.8121) ccw projected
  line L24 (-15.9432, -45.8121) -> (-69.7443, -45.8121) projected
  line L25 (158.214, -24.1186) -> (152.9786, -18.8832) projected
  arc A37 (160.0497, -1.8121) -> (152.9786, -18.8832) centre (160.0497, -11.8121) ccw projected
  line L26 (160.0497, -1.8121) -> (173.7802, -1.8121) projected
  arc A38 (178.72, -7.5859) -> (173.7802, -1.8121) centre (173.7802, -6.8121) ccw projected
  arc A39 (174.2037, -21.5706) -> (178.72, -7.5859) centre (132.2862, -0.3121) ccw projected
  arc A40 (158.214, -24.1186) -> (174.2037, -21.5706) centre (165.2851, -17.0475) ccw projected
  arc A41 (95.0878, 34.2305) -> (86.7862, 30.4755) centre (91.7862, 30.4755) ccw projected
  arc A42 (115.908, 12.7841) -> (95.0878, 34.2305) centre (-30.0061, -108.0406) ccw projected
  arc A43 (117.838, 3.7189) -> (115.908, 12.7841) centre (108.2059, 6.4063) ccw projected
  arc A44 (117.838, 3.7189) -> (117.837, -4.3395) centre (132.2862, -0.3121) ccw projected
  arc A45 (115.9016, -13.4079) -> (117.837, -4.3395) centre (108.2042, -7.0244) ccw projected
  arc A46 (95.0899, -34.8414) -> (115.9016, -13.4079) centre (-31.0421, 108.4524) ccw projected
  arc A47 (86.7862, -31.0883) -> (95.0899, -34.8414) centre (91.7862, -31.0883) ccw projected
  line L27 (86.7862, -31.0883) -> (86.7862, 30.4755) projected
  arc A48 (174.2862, 1.1879) -> (179.2862, 6.1879) centre (174.2862, 6.1879) ccw projected
  line L28 (174.2862, 1.1879) -> (160.4818, 1.1879) projected
  arc A49 (153.0118, 17.836) -> (160.4818, 1.1879) centre (160.4818, 11.1879) ccw projected
  arc A50 (171.0229, 35.5585) -> (153.0118, 17.836) centre (295.6146, -109.0766) ccw projected
  arc A51 (179.2862, 31.7702) -> (171.0229, 35.5585) centre (174.2862, 31.7702) ccw projected
  line L29 (179.2862, 31.7702) -> (179.2862, 6.1879) projected
  line L30 (-11.3182, -34.0226) -> (-36.0889, -7.0803) projected
  arc A52 (-36.0889, 6.4561) -> (-36.0889, -7.0803) centre (-28.7274, -0.3121) ccw projected
  line L31 (-36.0889, 6.4561) -> (-11.3182, 33.3984) projected
  arc A53 (-2.6374, 30.0143) -> (-11.3182, 33.3984) centre (-7.6374, 30.0143) ccw projected
  line L32 (-2.6374, 30.0143) -> (-2.6374, -30.6385) projected
  arc A54 (-11.3182, -34.0226) -> (-2.6374, -30.6385) centre (-7.6374, -30.6385) ccw projected
  line L33 (-158.3675, -26.2399) -> (-153.1321, -21.0045) projected
  arc A55 (-136.0611, -28.0756) -> (-153.1321, -21.0045) centre (-146.0611, -28.0756) ccw projected
  line L34 (-136.0611, -28.0756) -> (-136.0611, -41.8061) projected
  arc A56 (-141.8349, -46.7458) -> (-136.0611, -41.8061) centre (-141.0611, -41.8061) ccw projected
  arc A57 (-155.8196, -42.2296) -> (-141.8349, -46.7458) centre (-134.5611, -0.3121) ccw projected
  arc A58 (-158.3675, -26.2399) -> (-155.8196, -42.2296) centre (-151.2965, -33.311) ccw projected
  arc A59 (-120.1118, -4.3395) -> (-120.1128, 3.7189) centre (-134.5611, -0.3121) ccw projected
  arc A60 (-118.1829, 12.7841) -> (-120.1128, 3.7189) centre (-110.4807, 6.4063) ccw projected
  arc A61 (-97.3626, 34.2305) -> (-118.1829, 12.7841) centre (27.7313, -108.0406) ccw projected
  arc A62 (-89.0611, 30.4755) -> (-97.3626, 34.2305) centre (-94.0611, 30.4755) ccw projected
  line L35 (-89.0611, 30.4755) -> (-89.0611, -31.0883) projected
  arc A63 (-97.3647, -34.8414) -> (-89.0611, -31.0883) centre (-94.0611, -31.0883) ccw projected
  arc A64 (-118.1765, -13.4079) -> (-97.3647, -34.8414) centre (28.7673, 108.4524) ccw projected
  arc A65 (-120.1118, -4.3395) -> (-118.1765, -13.4079) centre (-110.479, -7.0244) ccw projected
  arc A66 (-102.4787, -47.3121) -> (-98.6905, -39.0488) centre (-102.4787, -42.3121) ccw projected
  line L36 (-102.4787, -47.3121) -> (-128.0611, -47.3121) projected
  arc A67 (-133.0611, -42.3121) -> (-128.0611, -47.3121) centre (-128.0611, -42.3121) ccw projected
  line L37 (-133.0611, -42.3121) -> (-133.0611, -28.5077) projected
  arc A68 (-116.4129, -21.0376) -> (-133.0611, -28.5077) centre (-123.0611, -28.5077) ccw projected
  arc A69 (-98.6905, -39.0488) -> (-116.4129, -21.0376) centre (-243.3255, -163.6405) ccw projected
  arc A70 (-74.1343, 46.6879) -> (-77.8151, 38.3038) centre (-74.1343, 41.6879) ccw projected
  line L38 (-74.1343, 46.6879) -> (-14.5641, 46.6879) projected
  arc A71 (-10.8834, 38.3038) -> (-14.5641, 46.6879) centre (-14.5641, 41.6879) ccw projected
  line L39 (-10.8834, 38.3038) -> (-36.9877, 9.911) projected
  arc A72 (-51.7107, 9.911) -> (-36.9877, 9.911) centre (-44.3492, 16.6792) ccw projected
  line L40 (-51.7107, 9.911) -> (-77.8151, 38.3038) projected
  arc A73 (130.7862, -28.5077) -> (114.1381, -21.0376) centre (120.7862, -28.5077) ccw projected
  line L41 (130.7862, -28.5077) -> (130.7862, -42.3121) projected
  arc A74 (125.7862, -47.3121) -> (130.7862, -42.3121) centre (125.7862, -42.3121) ccw projected
  line L42 (125.7862, -47.3121) -> (100.2039, -47.3121) projected
  arc A75 (96.4156, -39.0488) -> (100.2039, -47.3121) centre (100.2039, -42.3121) ccw projected
  arc A76 (114.1381, -21.0376) -> (96.4156, -39.0488) centre (241.0507, -163.6405) ccw projected
  line L43 (75.5403, 38.3038) -> (42.0744, 1.9041) projected
  line L44 (42.0744, 1.9041) -> (8.6085, 38.3038) projected
  arc A77 (12.2893, 46.6879) -> (8.6085, 38.3038) centre (12.2893, 41.6879) ccw projected
  line L45 (12.2893, 46.6879) -> (71.8595, 46.6879) projected
  arc A78 (75.5403, 38.3038) -> (71.8595, 46.6879) centre (71.8595, 41.6879) ccw projected
  line L46 (179.2862, 51.6879) -> (-181.5611, 51.6879) projected
  arc A79 (-181.5611, 51.6879) -> (-186.5611, 46.6879) centre (-181.5611, 46.6879) ccw projected
  line L47 (-186.5611, 46.6879) -> (-186.5611, -0.3121) projected
  arc A80 (-186.5611, -0.3121) -> (-134.5611, -52.3121) centre (-134.5611, -0.3121) ccw projected
  line L48 (-134.5611, -52.3121) -> (132.2862, -52.3121) projected
  arc A81 (132.2862, -52.3121) -> (184.2862, -0.3121) centre (132.2862, -0.3121) ccw projected
  line L49 (184.2862, -0.3121) -> (184.2862, 46.6879) projected
  arc A82 (184.2862, 46.6879) -> (179.2862, 51.6879) centre (179.2862, 46.6879) ccw projected
  circle A83 centre (85.2862, -47.3121) radius 2.1 projected
  circle A84 centre (179.2862, 46.6879) radius 2.1 projected
  circle A85 centre (85.2862, 46.6879) radius 2.1 projected
  circle A86 centre (-1.1374, 46.6879) radius 2.1 projected
  circle A87 centre (-87.5611, 46.6879) radius 2.1 projected
  circle A88 centre (-181.5611, 46.6879) radius 2.1 projected
  circle A89 centre (-87.5611, -47.3121) radius 2.1 projected
  circle A90 centre (123.2862, -0.3121) radius 2.1 projected
  circle A91 centre (132.2862, 8.6879) radius 2.1 projected
  circle A92 centre (-125.5611, -0.3121) radius 2.1 projected
  circle A93 centre (-134.5611, -9.3121) radius 2.1 projected
  circle A94 centre (-134.5611, 8.6879) radius 2.1 projected
  circle A95 centre (-1.1374, -47.3121) radius 2.1 projected
  circle A96 centre (132.2862, -0.3121) radius 4 projected
  circle A97 centre (132.2862, -9.3121) radius 2.1 projected
  circle A98 centre (141.2862, -0.3121) radius 2.1 projected
  circle A99 centre (-143.5611, -0.3121) radius 2.1 projected
  circle A100 centre (-134.5611, -0.3121) radius 4 projected
  point P0 (0, 0)
  point P1 (34.2021, -45.8121)
  point P2 (38.2774, -45.8121)
  point P3 (83.7862, 3.6863)
  point P4 (83.7862, 8.1188)
  point P5 (-36.4769, -45.8121)
  point P6 (-86.0611, 8.1188)
  point P7 (-86.0611, 3.6863)
  point P8 (-40.5522, -45.8121)
  dimension "d92" = 25
  dimension "d93" = 1.5
  dimension "d94" = 1.5
  constraints: 14 end point, 6 symmetric about line, 3 parallel, 1 vertical
  measures "d92" distance between parallel lines of L0 L1
  measures "d93" distance between parallel lines of L1 L2
  measures "d94" distance between parallel lines of L1 L3
extrude "Выдавливание4" add sketch "Эскиз6" against normal blind 2 contours L2 L24 L1 L22 | L1 L24 L3 L22 | L6 L15 L5 L16 | L5 L15 L7 L16
fillet "Сопряжение4" radius 10 9 edges at (-86.0611, 8.1188, 1) (-36.4769, -45.8121, 1) (-40.5522, -45.8121, 1) (34.2021, -45.8121, 1) (-86.0611, 3.6863, 1) (38.2774, -45.8121, 1) (83.7862, 8.1188, 1) (83.7862, 3.6863, 1) (42.0744, 1.9041, 1)
sketch "Эскиз7" plane through (0, 0, 2) normal (0, 0, 1) x (1, 0, 0)
  arc A0 (-15.9432, -45.8121) -> (-12.2625, -37.428) centre (-15.9432, -40.8121) ccw projected
  arc A1 (-77.3803, 33.3984) -> (-86.0611, 30.0143) centre (-81.0611, 30.0143) ccw projected
  arc A2 (-15.9432, -45.8121) -> (-86.0611, 30.0143) centre (-162.6046, -111.0994) ccw
  line L0 (-12.2625, -37.428) -> (-77.3803, 33.3984) projected
  arc A3 (83.7862, 30.0143) -> (75.1055, 33.3984) centre (78.7862, 30.0143) ccw projected
  arc A4 (9.9876, -37.428) -> (13.6684, -45.8121) centre (13.6684, -40.8121) ccw projected
  arc A5 (83.7862, 30.0143) -> (13.6684, -45.8121) centre (160.3298, -111.0994) ccw
  line L1 (75.1055, 33.3984) -> (9.9876, -37.428) projected
  point P0 (0, 0)
  point P1 (-44.4255, -2.4455)
  point P2 (42.1506, -2.4455)
  constraints: 4 point on circle, 2 centre point, 2 tangent
extrude "Выдавливание5" add sketch "Эскиз7" against normal blind 2
fillet "Сопряжение5" radius 10 4 edges at (83.7862, 30.0143, 1) (13.6684, -45.8121, 1) (-86.0611, 30.0143, 1) (-15.9432, -45.8121, 1)